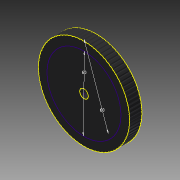
# Autodesk Inventor part: wheel 1
Saved by Autodesk Inventor 2014 (Build 180170000, 170)
## iProperties
Created: 2014-11-30
Part Number: wheel 1
Material: Generic
Document SubType Name: Modeling
Designer: ph1140784
Density: 1 g/cm^3
Appearance: Rubber - Black
Mass: 42.4685 g
Surface Area: 111.398 cm^2
Volume: 42.4685 cm^3
d0: 74.000 mm
d1: 10.000 mm
d2: 0.00 deg
d3: 7.000 mm
d4: 10.000 mm
d5: 0.00 deg
d7: 10.000 mm
d8: 0.00 deg
d9: 80.000 ul
d10: 360.00 deg
Author: ph1140784
Autodesk Inventor part; units mm, degrees
ref_plane "YZ Plane" through (0, 0, 0) normal (1, 0, 0) x (0, 1, 0)
ref_plane "XZ Plane" through (0, 0, 0) normal (0, 1, 0) x (-1, 0, 0)
ref_plane "XY Plane" through (0, 0, 0) normal (0, 0, 1) x (1, 0, 0)
sketch "Sketch1" plane through (0, 0, 0) normal (0, 1, 0) x (-1, 0, 0)
  circle A0 centre (0, 0) radius 37
  dimension "d0" = 74
  constraints: 1 centre point, 1 coincident
  measures "d0" diameter of A0
extrude "Extrusion1" add sketch "Sketch1" along normal blind 10
sketch "Sketch2" plane through (0, 10, 0) normal (0, 1, 0) x (1, 0, 0)
  circle A0 centre (0, 0) radius 37 projected
  circle A1 centre (0, 0) radius 3.5
  dimension "d3" = 7
  constraints: 1 centre point, 1 coincident
  measures "d3" diameter of A1
extrude "Extrusion2" cut sketch "Sketch2" against normal blind 10 contours A1
sketch "Sketch3" plane through (0, 10, 0) normal (0, 1, 0) x (1, 0, 0)
  circle A0 centre (0, 0) radius 37 projected
  line L0 (-16.7028, 33.0154) -> (-16.0314, 33.0154)
  line L1 (-16.0314, 33.0154) -> (-15.5404, 33.5782)
  constraints: 4 end point, 2 point on circle, 1 horizontal
extrude "Extrusion3" cut sketch "Sketch3" against normal blind 10 contours L1 L0 A0 picked at (-15.8339, 33.3296)
pattern_circular "Circular Pattern1" count 80 over 360 about axis through (0, -10, 0) along (0, 1, 0) of "Extrusion3"
sketch "Sketch4" plane through (0, 0, 0) normal (0, -1, 0) x (1, 0, 0)
  line L0 (-13.3916, -34.1714) -> (-12.858, -34.694) projected
  arc A0 (-12.858, -34.694) -> (-11.3324, -35.2218) centre (0, 0) ccw projected
  line L1 (-11.3324, -35.2218) -> (-10.6693, -35.1168) projected
  line L2 (-10.6693, -35.1168) -> (-10.0963, -35.5958) projected
  arc A1 (-10.0963, -35.5958) -> (-8.534, -36.0024) centre (0, 0) ccw projected
  line L3 (-8.534, -36.0024) -> (-7.8812, -35.8456) projected
  line L4 (-7.8812, -35.8456) -> (-7.2724, -36.2783) projected
  arc A2 (-7.2724, -36.2783) -> (-5.683, -36.561) centre (0, 0) ccw projected
  line L5 (-5.683, -36.561) -> (-5.0445, -36.3535) projected
  line L6 (-5.0445, -36.3535) -> (-4.4036, -36.737) projected
  arc A3 (-4.4036, -36.737) -> (-2.797, -36.8941) centre (0, 0) ccw projected
  line L7 (-2.797, -36.8941) -> (-2.1767, -36.6372) projected
  line L8 (-2.1767, -36.6372) -> (-1.5077, -36.9693) projected
  arc A4 (-1.5077, -36.9693) -> (0.1063, -36.9998) centre (0, 0) ccw projected
  line L9 (0.1063, -36.9998) -> (0.7046, -36.695) projected
  line L10 (0.7046, -36.695) -> (1.3976, -36.9736) projected
  arc A5 (1.3976, -36.9736) -> (3.009, -36.8774) centre (0, 0) ccw projected
  line L11 (3.009, -36.8774) -> (3.5815, -36.5266) projected
  line L12 (3.5815, -36.5266) -> (4.2942, -36.75) projected
  arc A6 (4.2942, -36.75) -> (5.8931, -36.5277) centre (0, 0) ccw projected
  line L13 (5.8931, -36.5277) -> (6.4363, -36.133) projected
  line L14 (6.4363, -36.133) -> (7.1643, -36.2998) projected
  arc A7 (7.1643, -36.2998) -> (8.7408, -35.9527) centre (0, 0) ccw projected
  line L15 (8.7408, -35.9527) -> (9.2514, -35.5167) projected
  line L16 (9.2514, -35.5167) -> (9.9903, -35.6258) projected
  arc A8 (9.9903, -35.6258) -> (11.5347, -35.1561) centre (0, 0) ccw projected
  line L17 (11.5347, -35.1561) -> (12.0095, -34.6813) projected
  line L18 (12.0095, -34.6813) -> (12.7546, -34.7321) projected
  arc A9 (12.7546, -34.7321) -> (14.2575, -34.1427) centre (0, 0) ccw projected
  line L19 (14.2575, -34.1427) -> (14.6935, -33.6322) projected
  line L20 (14.6935, -33.6322) -> (15.4404, -33.6243) projected
  arc A10 (15.4404, -33.6243) -> (16.8923, -32.9188) centre (0, 0) ccw projected
  line L21 (16.8923, -32.9188) -> (17.287, -32.3757) projected
  line L22 (17.287, -32.3757) -> (18.0309, -32.3092) projected
  arc A11 (18.0309, -32.3092) -> (19.423, -31.492) centre (0, 0) ccw projected
  line L23 (19.423, -31.492) -> (19.7738, -30.9195) projected
  line L24 (19.7738, -30.9195) -> (20.5103, -30.795) projected
  arc A12 (20.5103, -30.795) -> (21.834, -29.871) centre (0, 0) ccw projected
  line L25 (21.834, -29.871) -> (22.1388, -29.2728) projected
  line L26 (22.1388, -29.2728) -> (22.8632, -29.0908) projected
  arc A13 (22.8632, -29.0908) -> (24.1103, -28.0658) centre (0, 0) ccw projected
  line L27 (24.1103, -28.0658) -> (24.3673, -27.4455) projected
  line L28 (24.3673, -27.4455) -> (25.0751, -27.2073) projected
  arc A14 (25.0751, -27.2073) -> (26.238, -26.0876) centre (0, 0) ccw projected
  line L29 (26.238, -26.0876) -> (26.4455, -25.4491) projected
  line L30 (26.4455, -25.4491) -> (27.1325, -25.1561) projected
  arc A15 (27.1325, -25.1561) -> (28.204, -23.9486) centre (0, 0) ccw projected
  line L31 (28.204, -23.9486) -> (28.3607, -23.2958) projected
  line L32 (28.3607, -23.2958) -> (29.0226, -22.9497) projected
  arc A16 (29.0226, -22.9497) -> (29.996, -21.6619) centre (0, 0) ccw projected
  line L33 (29.996, -21.6619) -> (30.101, -20.9988) projected
  line L34 (30.101, -20.9988) -> (30.7337, -20.6019) projected
  arc A17 (30.7337, -20.6019) -> (31.6031, -19.2417) centre (0, 0) ccw projected
  line L35 (31.6031, -19.2417) -> (31.6558, -18.5724) projected
  line L36 (31.6558, -18.5724) -> (32.2554, -18.127) projected
  arc A18 (32.2554, -18.127) -> (33.0154, -16.7028) centre (0, 0) ccw projected
  line L37 (33.0154, -16.7028) -> (33.0154, -16.0314) projected
  line L38 (33.0154, -16.0314) -> (33.5782, -15.5404) projected
  arc A19 (33.5782, -15.5404) -> (34.2241, -14.061) centre (0, 0) ccw projected
  line L39 (34.2241, -14.061) -> (34.1714, -13.3916) projected
  line L40 (34.1714, -13.3916) -> (34.694, -12.858) projected
  arc A20 (34.694, -12.858) -> (35.2218, -11.3324) centre (0, 0) ccw projected
  line L41 (35.2218, -11.3324) -> (35.1168, -10.6693) projected
  line L42 (35.1168, -10.6693) -> (35.5958, -10.0963) projected
  arc A21 (35.5958, -10.0963) -> (36.0024, -8.534) centre (0, 0) ccw projected
  line L43 (36.0024, -8.534) -> (35.8456, -7.8812) projected
  line L44 (35.8456, -7.8812) -> (36.2783, -7.2724) projected
  arc A22 (36.2783, -7.2724) -> (36.561, -5.683) centre (0, 0) ccw projected
  line L45 (36.561, -5.683) -> (36.3535, -5.0445) projected
  line L46 (36.3535, -5.0445) -> (36.737, -4.4036) projected
  arc A23 (36.737, -4.4036) -> (36.8941, -2.797) centre (0, 0) ccw projected
  line L47 (36.8941, -2.797) -> (36.6372, -2.1767) projected
  line L48 (36.6372, -2.1767) -> (36.9693, -1.5077) projected
  arc A24 (36.9693, -1.5077) -> (36.9998, 0.1063) centre (0, 0) ccw projected
  line L49 (36.9998, 0.1063) -> (36.695, 0.7046) projected
  line L50 (36.695, 0.7046) -> (36.9736, 1.3976) projected
  arc A25 (36.9736, 1.3976) -> (36.8774, 3.009) centre (0, 0) ccw projected
  line L51 (36.8774, 3.009) -> (36.5266, 3.5815) projected
  line L52 (36.5266, 3.5815) -> (36.75, 4.2942) projected
  arc A26 (36.75, 4.2942) -> (36.5277, 5.8931) centre (0, 0) ccw projected
  line L53 (36.5277, 5.8931) -> (36.133, 6.4363) projected
  line L54 (36.133, 6.4363) -> (36.2998, 7.1643) projected
  arc A27 (36.2998, 7.1643) -> (35.9527, 8.7408) centre (0, 0) ccw projected
  line L55 (35.9527, 8.7408) -> (35.5167, 9.2514) projected
  line L56 (35.5167, 9.2514) -> (35.6258, 9.9903) projected
  arc A28 (35.6258, 9.9903) -> (35.1561, 11.5347) centre (0, 0) ccw projected
  line L57 (35.1561, 11.5347) -> (34.6813, 12.0095) projected
  line L58 (34.6813, 12.0095) -> (34.7321, 12.7546) projected
  arc A29 (34.7321, 12.7546) -> (34.1427, 14.2575) centre (0, 0) ccw projected
  line L59 (34.1427, 14.2575) -> (33.6322, 14.6935) projected
  line L60 (33.6322, 14.6935) -> (33.6243, 15.4404) projected
  arc A30 (33.6243, 15.4404) -> (32.9188, 16.8923) centre (0, 0) ccw projected
  line L61 (32.9188, 16.8923) -> (32.3757, 17.287) projected
  line L62 (32.3757, 17.287) -> (32.3092, 18.0309) projected
  arc A31 (32.3092, 18.0309) -> (31.492, 19.423) centre (0, 0) ccw projected
  line L63 (31.492, 19.423) -> (30.9195, 19.7738) projected
  line L64 (30.9195, 19.7738) -> (30.795, 20.5103) projected
  arc A32 (30.795, 20.5103) -> (29.871, 21.834) centre (0, 0) ccw projected
  line L65 (29.871, 21.834) -> (29.2728, 22.1388) projected
  line L66 (29.2728, 22.1388) -> (29.0908, 22.8632) projected
  arc A33 (29.0908, 22.8632) -> (28.0658, 24.1103) centre (0, 0) ccw projected
  line L67 (28.0658, 24.1103) -> (27.4455, 24.3673) projected
  line L68 (27.4455, 24.3673) -> (27.2073, 25.0751) projected
  arc A34 (27.2073, 25.0751) -> (26.0876, 26.238) centre (0, 0) ccw projected
  line L69 (26.0876, 26.238) -> (25.4491, 26.4455) projected
  line L70 (25.4491, 26.4455) -> (25.1561, 27.1325) projected
  arc A35 (25.1561, 27.1325) -> (23.9486, 28.204) centre (0, 0) ccw projected
  line L71 (23.9486, 28.204) -> (23.2958, 28.3607) projected
  line L72 (23.2958, 28.3607) -> (22.9497, 29.0226) projected
  arc A36 (22.9497, 29.0226) -> (21.6619, 29.996) centre (0, 0) ccw projected
  line L73 (21.6619, 29.996) -> (20.9988, 30.101) projected
  line L74 (20.9988, 30.101) -> (20.6019, 30.7337) projected
  arc A37 (20.6019, 30.7337) -> (19.2417, 31.6031) centre (0, 0) ccw projected
  line L75 (19.2417, 31.6031) -> (18.5724, 31.6558) projected
  line L76 (18.5724, 31.6558) -> (18.127, 32.2554) projected
  arc A38 (18.127, 32.2554) -> (16.7028, 33.0154) centre (0, 0) ccw projected
  line L77 (16.7028, 33.0154) -> (16.0314, 33.0154) projected
  line L78 (16.0314, 33.0154) -> (15.5404, 33.5782) projected
  arc A39 (15.5404, 33.5782) -> (14.061, 34.2241) centre (0, 0) ccw projected
  line L79 (14.061, 34.2241) -> (13.3916, 34.1714) projected
  line L80 (13.3916, 34.1714) -> (12.858, 34.694) projected
  arc A40 (12.858, 34.694) -> (11.3324, 35.2218) centre (0, 0) ccw projected
  line L81 (11.3324, 35.2218) -> (10.6693, 35.1168) projected
  line L82 (10.6693, 35.1168) -> (10.0963, 35.5958) projected
  arc A41 (10.0963, 35.5958) -> (8.534, 36.0024) centre (0, 0) ccw projected
  line L83 (8.534, 36.0024) -> (7.8812, 35.8456) projected
  line L84 (7.8812, 35.8456) -> (7.2724, 36.2783) projected
  arc A42 (7.2724, 36.2783) -> (5.683, 36.561) centre (0, 0) ccw projected
  line L85 (5.683, 36.561) -> (5.0445, 36.3535) projected
  line L86 (5.0445, 36.3535) -> (4.4036, 36.737) projected
  arc A43 (4.4036, 36.737) -> (2.797, 36.8941) centre (0, 0) ccw projected
  line L87 (2.797, 36.8941) -> (2.1767, 36.6372) projected
  line L88 (2.1767, 36.6372) -> (1.5077, 36.9693) projected
  arc A44 (1.5077, 36.9693) -> (-0.1063, 36.9998) centre (0, 0) ccw projected
  line L89 (-0.1063, 36.9998) -> (-0.7046, 36.695) projected
  line L90 (-0.7046, 36.695) -> (-1.3976, 36.9736) projected
  arc A45 (-1.3976, 36.9736) -> (-3.009, 36.8774) centre (0, 0) ccw projected
  line L91 (-3.009, 36.8774) -> (-3.5815, 36.5266) projected
  line L92 (-3.5815, 36.5266) -> (-4.2942, 36.75) projected
  arc A46 (-4.2942, 36.75) -> (-5.8931, 36.5277) centre (0, 0) ccw projected
  line L93 (-5.8931, 36.5277) -> (-6.4363, 36.133) projected
  line L94 (-6.4363, 36.133) -> (-7.1643, 36.2998) projected
  arc A47 (-7.1643, 36.2998) -> (-8.7408, 35.9527) centre (0, 0) ccw projected
  line L95 (-8.7408, 35.9527) -> (-9.2514, 35.5167) projected
  line L96 (-9.2514, 35.5167) -> (-9.9903, 35.6258) projected
  arc A48 (-9.9903, 35.6258) -> (-11.5347, 35.1561) centre (0, 0) ccw projected
  line L97 (-11.5347, 35.1561) -> (-12.0095, 34.6813) projected
  line L98 (-12.0095, 34.6813) -> (-12.7546, 34.7321) projected
  arc A49 (-12.7546, 34.7321) -> (-14.2575, 34.1427) centre (0, 0) ccw projected
  line L99 (-14.2575, 34.1427) -> (-14.6935, 33.6322) projected
  line L100 (-14.6935, 33.6322) -> (-15.4404, 33.6243) projected
  arc A50 (-15.4404, 33.6243) -> (-16.8923, 32.9188) centre (0, 0) ccw projected
  line L101 (-16.8923, 32.9188) -> (-17.287, 32.3757) projected
  line L102 (-17.287, 32.3757) -> (-18.0309, 32.3092) projected
  arc A51 (-18.0309, 32.3092) -> (-19.423, 31.492) centre (0, 0) ccw projected
  line L103 (-19.423, 31.492) -> (-19.7738, 30.9195) projected
  line L104 (-19.7738, 30.9195) -> (-20.5103, 30.795) projected
  arc A52 (-20.5103, 30.795) -> (-21.834, 29.871) centre (0, 0) ccw projected
  line L105 (-21.834, 29.871) -> (-22.1388, 29.2728) projected
  line L106 (-22.1388, 29.2728) -> (-22.8632, 29.0908) projected
  arc A53 (-22.8632, 29.0908) -> (-24.1103, 28.0658) centre (0, 0) ccw projected
  line L107 (-24.1103, 28.0658) -> (-24.3673, 27.4455) projected
  line L108 (-24.3673, 27.4455) -> (-25.0751, 27.2073) projected
  arc A54 (-25.0751, 27.2073) -> (-26.238, 26.0876) centre (0, 0) ccw projected
  line L109 (-26.238, 26.0876) -> (-26.4455, 25.4491) projected
  line L110 (-26.4455, 25.4491) -> (-27.1325, 25.1561) projected
  arc A55 (-27.1325, 25.1561) -> (-28.204, 23.9486) centre (0, 0) ccw projected
  line L111 (-28.204, 23.9486) -> (-28.3607, 23.2958) projected
  line L112 (-28.3607, 23.2958) -> (-29.0226, 22.9497) projected
  arc A56 (-29.0226, 22.9497) -> (-29.996, 21.6619) centre (0, 0) ccw projected
  line L113 (-29.996, 21.6619) -> (-30.101, 20.9988) projected
  line L114 (-30.101, 20.9988) -> (-30.7337, 20.6019) projected
  arc A57 (-30.7337, 20.6019) -> (-31.6031, 19.2417) centre (0, 0) ccw projected
  line L115 (-31.6031, 19.2417) -> (-31.6558, 18.5724) projected
  line L116 (-31.6558, 18.5724) -> (-32.2554, 18.127) projected
  arc A58 (-32.2554, 18.127) -> (-33.0154, 16.7028) centre (0, 0) ccw projected
  line L117 (-33.0154, 16.7028) -> (-33.0154, 16.0314) projected
  line L118 (-33.0154, 16.0314) -> (-33.5782, 15.5404) projected
  arc A59 (-33.5782, 15.5404) -> (-34.2241, 14.061) centre (0, 0) ccw projected
  line L119 (-34.2241, 14.061) -> (-34.1714, 13.3916) projected
  line L120 (-34.1714, 13.3916) -> (-34.694, 12.858) projected
  arc A60 (-34.694, 12.858) -> (-35.2218, 11.3324) centre (0, 0) ccw projected
  line L121 (-35.2218, 11.3324) -> (-35.1168, 10.6693) projected
  line L122 (-35.1168, 10.6693) -> (-35.5958, 10.0963) projected
  arc A61 (-35.5958, 10.0963) -> (-36.0024, 8.534) centre (0, 0) ccw projected
  line L123 (-36.0024, 8.534) -> (-35.8456, 7.8812) projected
  line L124 (-35.8456, 7.8812) -> (-36.2783, 7.2724) projected
  arc A62 (-36.2783, 7.2724) -> (-36.561, 5.683) centre (0, 0) ccw projected
  line L125 (-36.561, 5.683) -> (-36.3535, 5.0445) projected
  line L126 (-36.3535, 5.0445) -> (-36.737, 4.4036) projected
  arc A63 (-36.737, 4.4036) -> (-36.8941, 2.797) centre (0, 0) ccw projected
  line L127 (-36.8941, 2.797) -> (-36.6372, 2.1767) projected
  line L128 (-36.6372, 2.1767) -> (-36.9693, 1.5077) projected
  arc A64 (-36.9693, 1.5077) -> (-36.9998, -0.1063) centre (0, 0) ccw projected
  line L129 (-36.9998, -0.1063) -> (-36.695, -0.7046) projected
  line L130 (-36.695, -0.7046) -> (-36.9736, -1.3976) projected
  arc A65 (-36.9736, -1.3976) -> (-36.8774, -3.009) centre (0, 0) ccw projected
  line L131 (-36.8774, -3.009) -> (-36.5266, -3.5815) projected
  line L132 (-36.5266, -3.5815) -> (-36.75, -4.2942) projected
  arc A66 (-36.75, -4.2942) -> (-36.5277, -5.8931) centre (0, 0) ccw projected
  line L133 (-36.5277, -5.8931) -> (-36.133, -6.4363) projected
  line L134 (-36.133, -6.4363) -> (-36.2998, -7.1643) projected
  arc A67 (-36.2998, -7.1643) -> (-35.9527, -8.7408) centre (0, 0) ccw projected
  line L135 (-35.9527, -8.7408) -> (-35.5167, -9.2514) projected
  line L136 (-35.5167, -9.2514) -> (-35.6258, -9.9903) projected
  arc A68 (-35.6258, -9.9903) -> (-35.1561, -11.5347) centre (0, 0) ccw projected
  line L137 (-35.1561, -11.5347) -> (-34.6813, -12.0095) projected
  line L138 (-34.6813, -12.0095) -> (-34.7321, -12.7546) projected
  arc A69 (-34.7321, -12.7546) -> (-34.1427, -14.2575) centre (0, 0) ccw projected
  line L139 (-34.1427, -14.2575) -> (-33.6322, -14.6935) projected
  line L140 (-33.6322, -14.6935) -> (-33.6243, -15.4404) projected
  arc A70 (-33.6243, -15.4404) -> (-32.9188, -16.8923) centre (0, 0) ccw projected
  line L141 (-32.9188, -16.8923) -> (-32.3757, -17.287) projected
  line L142 (-32.3757, -17.287) -> (-32.3092, -18.0309) projected
  arc A71 (-32.3092, -18.0309) -> (-31.492, -19.423) centre (0, 0) ccw projected
  line L143 (-31.492, -19.423) -> (-30.9195, -19.7738) projected
  line L144 (-30.9195, -19.7738) -> (-30.795, -20.5103) projected
  arc A72 (-30.795, -20.5103) -> (-29.871, -21.834) centre (0, 0) ccw projected
  line L145 (-29.871, -21.834) -> (-29.2728, -22.1388) projected
  line L146 (-29.2728, -22.1388) -> (-29.0908, -22.8632) projected
  arc A73 (-29.0908, -22.8632) -> (-28.0658, -24.1103) centre (0, 0) ccw projected
  line L147 (-28.0658, -24.1103) -> (-27.4455, -24.3673) projected
  line L148 (-27.4455, -24.3673) -> (-27.2073, -25.0751) projected
  arc A74 (-27.2073, -25.0751) -> (-26.0876, -26.238) centre (0, 0) ccw projected
  line L149 (-26.0876, -26.238) -> (-25.4491, -26.4455) projected
  line L150 (-25.4491, -26.4455) -> (-25.1561, -27.1325) projected
  arc A75 (-25.1561, -27.1325) -> (-23.9486, -28.204) centre (0, 0) ccw projected
  line L151 (-23.9486, -28.204) -> (-23.2958, -28.3607) projected
  line L152 (-23.2958, -28.3607) -> (-22.9497, -29.0226) projected
  arc A76 (-22.9497, -29.0226) -> (-21.6619, -29.996) centre (0, 0) ccw projected
  line L153 (-21.6619, -29.996) -> (-20.9988, -30.101) projected
  line L154 (-20.9988, -30.101) -> (-20.6019, -30.7337) projected
  arc A77 (-20.6019, -30.7337) -> (-19.2417, -31.6031) centre (0, 0) ccw projected
  line L155 (-19.2417, -31.6031) -> (-18.5724, -31.6558) projected
  line L156 (-18.5724, -31.6558) -> (-18.127, -32.2554) projected
  arc A78 (-18.127, -32.2554) -> (-16.7028, -33.0154) centre (0, 0) ccw projected
  line L157 (-16.7028, -33.0154) -> (-16.0314, -33.0154) projected
  line L158 (-16.0314, -33.0154) -> (-15.5404, -33.5782) projected
  arc A79 (-15.5404, -33.5782) -> (-14.061, -34.2241) centre (0, 0) ccw projected
  line L159 (-14.061, -34.2241) -> (-13.3916, -34.1714) projected
  circle A80 centre (0, 0) radius 3.5 projected
  circle A81 centre (0, 0) radius 30
  dimension "d12" = 60
  constraints: 1 centre point, 1 coincident
  measures "d12" diameter of A81
sketch "Sketch5" plane through (0, 10, 0) normal (0, 1, 0) x (1, 0, 0)
  circle A0 centre (0, 0) radius 3.5 projected
  line L0 (-12.858, 34.694) -> (-13.3916, 34.1714) projected
  line L1 (-13.3916, 34.1714) -> (-14.061, 34.2241) projected
  arc A1 (-14.061, 34.2241) -> (-15.5404, 33.5782) centre (0, 0) ccw projected
  line L2 (-15.5404, 33.5782) -> (-16.0314, 33.0154) projected
  line L3 (-16.0314, 33.0154) -> (-16.7028, 33.0154) projected
  arc A2 (-16.7028, 33.0154) -> (-18.127, 32.2554) centre (0, 0) ccw projected
  line L4 (-18.127, 32.2554) -> (-18.5724, 31.6558) projected
  line L5 (-18.5724, 31.6558) -> (-19.2417, 31.6031) projected
  arc A3 (-19.2417, 31.6031) -> (-20.6019, 30.7337) centre (0, 0) ccw projected
  line L6 (-20.6019, 30.7337) -> (-20.9988, 30.101) projected
  line L7 (-20.9988, 30.101) -> (-21.6619, 29.996) projected
  arc A4 (-21.6619, 29.996) -> (-22.9497, 29.0226) centre (0, 0) ccw projected
  line L8 (-22.9497, 29.0226) -> (-23.2958, 28.3607) projected
  line L9 (-23.2958, 28.3607) -> (-23.9486, 28.204) projected
  arc A5 (-23.9486, 28.204) -> (-25.1561, 27.1325) centre (0, 0) ccw projected
  line L10 (-25.1561, 27.1325) -> (-25.4491, 26.4455) projected
  line L11 (-25.4491, 26.4455) -> (-26.0876, 26.238) projected
  arc A6 (-26.0876, 26.238) -> (-27.2073, 25.0751) centre (0, 0) ccw projected
  line L12 (-27.2073, 25.0751) -> (-27.4455, 24.3673) projected
  line L13 (-27.4455, 24.3673) -> (-28.0658, 24.1103) projected
  arc A7 (-28.0658, 24.1103) -> (-29.0908, 22.8632) centre (0, 0) ccw projected
  line L14 (-29.0908, 22.8632) -> (-29.2728, 22.1388) projected
  line L15 (-29.2728, 22.1388) -> (-29.871, 21.834) projected
  arc A8 (-29.871, 21.834) -> (-30.795, 20.5103) centre (0, 0) ccw projected
  line L16 (-30.795, 20.5103) -> (-30.9195, 19.7738) projected
  line L17 (-30.9195, 19.7738) -> (-31.492, 19.423) projected
  arc A9 (-31.492, 19.423) -> (-32.3092, 18.0309) centre (0, 0) ccw projected
  line L18 (-32.3092, 18.0309) -> (-32.3757, 17.287) projected
  line L19 (-32.3757, 17.287) -> (-32.9188, 16.8923) projected
  arc A10 (-32.9188, 16.8923) -> (-33.6243, 15.4404) centre (0, 0) ccw projected
  line L20 (-33.6243, 15.4404) -> (-33.6322, 14.6935) projected
  line L21 (-33.6322, 14.6935) -> (-34.1427, 14.2575) projected
  arc A11 (-34.1427, 14.2575) -> (-34.7321, 12.7546) centre (0, 0) ccw projected
  line L22 (-34.7321, 12.7546) -> (-34.6813, 12.0095) projected
  line L23 (-34.6813, 12.0095) -> (-35.1561, 11.5347) projected
  arc A12 (-35.1561, 11.5347) -> (-35.6258, 9.9903) centre (0, 0) ccw projected
  line L24 (-35.6258, 9.9903) -> (-35.5167, 9.2514) projected
  line L25 (-35.5167, 9.2514) -> (-35.9527, 8.7408) projected
  arc A13 (-35.9527, 8.7408) -> (-36.2998, 7.1643) centre (0, 0) ccw projected
  line L26 (-36.2998, 7.1643) -> (-36.133, 6.4363) projected
  line L27 (-36.133, 6.4363) -> (-36.5277, 5.8931) projected
  arc A14 (-36.5277, 5.8931) -> (-36.75, 4.2942) centre (0, 0) ccw projected
  line L28 (-36.75, 4.2942) -> (-36.5266, 3.5815) projected
  line L29 (-36.5266, 3.5815) -> (-36.8774, 3.009) projected
  arc A15 (-36.8774, 3.009) -> (-36.9736, 1.3976) centre (0, 0) ccw projected
  line L30 (-36.9736, 1.3976) -> (-36.695, 0.7046) projected
  line L31 (-36.695, 0.7046) -> (-36.9998, 0.1063) projected
  arc A16 (-36.9998, 0.1063) -> (-36.9693, -1.5077) centre (0, 0) ccw projected
  line L32 (-36.9693, -1.5077) -> (-36.6372, -2.1767) projected
  line L33 (-36.6372, -2.1767) -> (-36.8941, -2.797) projected
  arc A17 (-36.8941, -2.797) -> (-36.737, -4.4036) centre (0, 0) ccw projected
  line L34 (-36.737, -4.4036) -> (-36.3535, -5.0445) projected
  line L35 (-36.3535, -5.0445) -> (-36.561, -5.683) projected
  arc A18 (-36.561, -5.683) -> (-36.2783, -7.2724) centre (0, 0) ccw projected
  line L36 (-36.2783, -7.2724) -> (-35.8456, -7.8812) projected
  line L37 (-35.8456, -7.8812) -> (-36.0024, -8.534) projected
  arc A19 (-36.0024, -8.534) -> (-35.5958, -10.0963) centre (0, 0) ccw projected
  line L38 (-35.5958, -10.0963) -> (-35.1168, -10.6693) projected
  line L39 (-35.1168, -10.6693) -> (-35.2218, -11.3324) projected
  arc A20 (-35.2218, -11.3324) -> (-34.694, -12.858) centre (0, 0) ccw projected
  line L40 (-34.694, -12.858) -> (-34.1714, -13.3916) projected
  line L41 (-34.1714, -13.3916) -> (-34.2241, -14.061) projected
  arc A21 (-34.2241, -14.061) -> (-33.5782, -15.5404) centre (0, 0) ccw projected
  line L42 (-33.5782, -15.5404) -> (-33.0154, -16.0314) projected
  line L43 (-33.0154, -16.0314) -> (-33.0154, -16.7028) projected
  arc A22 (-33.0154, -16.7028) -> (-32.2554, -18.127) centre (0, 0) ccw projected
  line L44 (-32.2554, -18.127) -> (-31.6558, -18.5724) projected
  line L45 (-31.6558, -18.5724) -> (-31.6031, -19.2417) projected
  arc A23 (-31.6031, -19.2417) -> (-30.7337, -20.6019) centre (0, 0) ccw projected
  line L46 (-30.7337, -20.6019) -> (-30.101, -20.9988) projected
  line L47 (-30.101, -20.9988) -> (-29.996, -21.6619) projected
  arc A24 (-29.996, -21.6619) -> (-29.0226, -22.9497) centre (0, 0) ccw projected
  line L48 (-29.0226, -22.9497) -> (-28.3607, -23.2958) projected
  line L49 (-28.3607, -23.2958) -> (-28.204, -23.9486) projected
  arc A25 (-28.204, -23.9486) -> (-27.1325, -25.1561) centre (0, 0) ccw projected
  line L50 (-27.1325, -25.1561) -> (-26.4455, -25.4491) projected
  line L51 (-26.4455, -25.4491) -> (-26.238, -26.0876) projected
  arc A26 (-26.238, -26.0876) -> (-25.0751, -27.2073) centre (0, 0) ccw projected
  line L52 (-25.0751, -27.2073) -> (-24.3673, -27.4455) projected
  line L53 (-24.3673, -27.4455) -> (-24.1103, -28.0658) projected
  arc A27 (-24.1103, -28.0658) -> (-22.8632, -29.0908) centre (0, 0) ccw projected
  line L54 (-22.8632, -29.0908) -> (-22.1388, -29.2728) projected
  line L55 (-22.1388, -29.2728) -> (-21.834, -29.871) projected
  arc A28 (-21.834, -29.871) -> (-20.5103, -30.795) centre (0, 0) ccw projected
  line L56 (-20.5103, -30.795) -> (-19.7738, -30.9195) projected
  line L57 (-19.7738, -30.9195) -> (-19.423, -31.492) projected
  arc A29 (-19.423, -31.492) -> (-18.0309, -32.3092) centre (0, 0) ccw projected
  line L58 (-18.0309, -32.3092) -> (-17.287, -32.3757) projected
  line L59 (-17.287, -32.3757) -> (-16.8923, -32.9188) projected
  arc A30 (-16.8923, -32.9188) -> (-15.4404, -33.6243) centre (0, 0) ccw projected
  line L60 (-15.4404, -33.6243) -> (-14.6935, -33.6322) projected
  line L61 (-14.6935, -33.6322) -> (-14.2575, -34.1427) projected
  arc A31 (-14.2575, -34.1427) -> (-12.7546, -34.7321) centre (0, 0) ccw projected
  line L62 (-12.7546, -34.7321) -> (-12.0095, -34.6813) projected
  line L63 (-12.0095, -34.6813) -> (-11.5347, -35.1561) projected
  arc A32 (-11.5347, -35.1561) -> (-9.9903, -35.6258) centre (0, 0) ccw projected
  line L64 (-9.9903, -35.6258) -> (-9.2514, -35.5167) projected
  line L65 (-9.2514, -35.5167) -> (-8.7408, -35.9527) projected
  arc A33 (-8.7408, -35.9527) -> (-7.1643, -36.2998) centre (0, 0) ccw projected
  line L66 (-7.1643, -36.2998) -> (-6.4363, -36.133) projected
  line L67 (-6.4363, -36.133) -> (-5.8931, -36.5277) projected
  arc A34 (-5.8931, -36.5277) -> (-4.2942, -36.75) centre (0, 0) ccw projected
  line L68 (-4.2942, -36.75) -> (-3.5815, -36.5266) projected
  line L69 (-3.5815, -36.5266) -> (-3.009, -36.8774) projected
  arc A35 (-3.009, -36.8774) -> (-1.3976, -36.9736) centre (0, 0) ccw projected
  line L70 (-1.3976, -36.9736) -> (-0.7046, -36.695) projected
  line L71 (-0.7046, -36.695) -> (-0.1063, -36.9998) projected
  arc A36 (-0.1063, -36.9998) -> (1.5077, -36.9693) centre (0, 0) ccw projected
  line L72 (1.5077, -36.9693) -> (2.1767, -36.6372) projected
  line L73 (2.1767, -36.6372) -> (2.797, -36.8941) projected
  arc A37 (2.797, -36.8941) -> (4.4036, -36.737) centre (0, 0) ccw projected
  line L74 (4.4036, -36.737) -> (5.0445, -36.3535) projected
  line L75 (5.0445, -36.3535) -> (5.683, -36.561) projected
  arc A38 (5.683, -36.561) -> (7.2724, -36.2783) centre (0, 0) ccw projected
  line L76 (7.2724, -36.2783) -> (7.8812, -35.8456) projected
  line L77 (7.8812, -35.8456) -> (8.534, -36.0024) projected
  arc A39 (8.534, -36.0024) -> (10.0963, -35.5958) centre (0, 0) ccw projected
  line L78 (10.0963, -35.5958) -> (10.6693, -35.1168) projected
  line L79 (10.6693, -35.1168) -> (11.3324, -35.2218) projected
  arc A40 (11.3324, -35.2218) -> (12.858, -34.694) centre (0, 0) ccw projected
  line L80 (12.858, -34.694) -> (13.3916, -34.1714) projected
  line L81 (13.3916, -34.1714) -> (14.061, -34.2241) projected
  arc A41 (14.061, -34.2241) -> (15.5404, -33.5782) centre (0, 0) ccw projected
  line L82 (15.5404, -33.5782) -> (16.0314, -33.0154) projected
  line L83 (16.0314, -33.0154) -> (16.7028, -33.0154) projected
  arc A42 (16.7028, -33.0154) -> (18.127, -32.2554) centre (0, 0) ccw projected
  line L84 (18.127, -32.2554) -> (18.5724, -31.6558) projected
  line L85 (18.5724, -31.6558) -> (19.2417, -31.6031) projected
  arc A43 (19.2417, -31.6031) -> (20.6019, -30.7337) centre (0, 0) ccw projected
  line L86 (20.6019, -30.7337) -> (20.9988, -30.101) projected
  line L87 (20.9988, -30.101) -> (21.6619, -29.996) projected
  arc A44 (21.6619, -29.996) -> (22.9497, -29.0226) centre (0, 0) ccw projected
  line L88 (22.9497, -29.0226) -> (23.2958, -28.3607) projected
  line L89 (23.2958, -28.3607) -> (23.9486, -28.204) projected
  arc A45 (23.9486, -28.204) -> (25.1561, -27.1325) centre (0, 0) ccw projected
  line L90 (25.1561, -27.1325) -> (25.4491, -26.4455) projected
  line L91 (25.4491, -26.4455) -> (26.0876, -26.238) projected
  arc A46 (26.0876, -26.238) -> (27.2073, -25.0751) centre (0, 0) ccw projected
  line L92 (27.2073, -25.0751) -> (27.4455, -24.3673) projected
  line L93 (27.4455, -24.3673) -> (28.0658, -24.1103) projected
  arc A47 (28.0658, -24.1103) -> (29.0908, -22.8632) centre (0, 0) ccw projected
  line L94 (29.0908, -22.8632) -> (29.2728, -22.1388) projected
  line L95 (29.2728, -22.1388) -> (29.871, -21.834) projected
  arc A48 (29.871, -21.834) -> (30.795, -20.5103) centre (0, 0) ccw projected
  line L96 (30.795, -20.5103) -> (30.9195, -19.7738) projected
  line L97 (30.9195, -19.7738) -> (31.492, -19.423) projected
  arc A49 (31.492, -19.423) -> (32.3092, -18.0309) centre (0, 0) ccw projected
  line L98 (32.3092, -18.0309) -> (32.3757, -17.287) projected
  line L99 (32.3757, -17.287) -> (32.9188, -16.8923) projected
  arc A50 (32.9188, -16.8923) -> (33.6243, -15.4404) centre (0, 0) ccw projected
  line L100 (33.6243, -15.4404) -> (33.6322, -14.6935) projected
  line L101 (33.6322, -14.6935) -> (34.1427, -14.2575) projected
  arc A51 (34.1427, -14.2575) -> (34.7321, -12.7546) centre (0, 0) ccw projected
  line L102 (34.7321, -12.7546) -> (34.6813, -12.0095) projected
  line L103 (34.6813, -12.0095) -> (35.1561, -11.5347) projected
  arc A52 (35.1561, -11.5347) -> (35.6258, -9.9903) centre (0, 0) ccw projected
  line L104 (35.6258, -9.9903) -> (35.5167, -9.2514) projected
  line L105 (35.5167, -9.2514) -> (35.9527, -8.7408) projected
  arc A53 (35.9527, -8.7408) -> (36.2998, -7.1643) centre (0, 0) ccw projected
  line L106 (36.2998, -7.1643) -> (36.133, -6.4363) projected
  line L107 (36.133, -6.4363) -> (36.5277, -5.8931) projected
  arc A54 (36.5277, -5.8931) -> (36.75, -4.2942) centre (0, 0) ccw projected
  line L108 (36.75, -4.2942) -> (36.5266, -3.5815) projected
  line L109 (36.5266, -3.5815) -> (36.8774, -3.009) projected
  arc A55 (36.8774, -3.009) -> (36.9736, -1.3976) centre (0, 0) ccw projected
  line L110 (36.9736, -1.3976) -> (36.695, -0.7046) projected
  line L111 (36.695, -0.7046) -> (36.9998, -0.1063) projected
  arc A56 (36.9998, -0.1063) -> (36.9693, 1.5077) centre (0, 0) ccw projected
  line L112 (36.9693, 1.5077) -> (36.6372, 2.1767) projected
  line L113 (36.6372, 2.1767) -> (36.8941, 2.797) projected
  arc A57 (36.8941, 2.797) -> (36.737, 4.4036) centre (0, 0) ccw projected
  line L114 (36.737, 4.4036) -> (36.3535, 5.0445) projected
  line L115 (36.3535, 5.0445) -> (36.561, 5.683) projected
  arc A58 (36.561, 5.683) -> (36.2783, 7.2724) centre (0, 0) ccw projected
  line L116 (36.2783, 7.2724) -> (35.8456, 7.8812) projected
  line L117 (35.8456, 7.8812) -> (36.0024, 8.534) projected
  arc A59 (36.0024, 8.534) -> (35.5958, 10.0963) centre (0, 0) ccw projected
  line L118 (35.5958, 10.0963) -> (35.1168, 10.6693) projected
  line L119 (35.1168, 10.6693) -> (35.2218, 11.3324) projected
  arc A60 (35.2218, 11.3324) -> (34.694, 12.858) centre (0, 0) ccw projected
  line L120 (34.694, 12.858) -> (34.1714, 13.3916) projected
  line L121 (34.1714, 13.3916) -> (34.2241, 14.061) projected
  arc A61 (34.2241, 14.061) -> (33.5782, 15.5404) centre (0, 0) ccw projected
  line L122 (33.5782, 15.5404) -> (33.0154, 16.0314) projected
  line L123 (33.0154, 16.0314) -> (33.0154, 16.7028) projected
  arc A62 (33.0154, 16.7028) -> (32.2554, 18.127) centre (0, 0) ccw projected
  line L124 (32.2554, 18.127) -> (31.6558, 18.5724) projected
  line L125 (31.6558, 18.5724) -> (31.6031, 19.2417) projected
  arc A63 (31.6031, 19.2417) -> (30.7337, 20.6019) centre (0, 0) ccw projected
  line L126 (30.7337, 20.6019) -> (30.101, 20.9988) projected
  line L127 (30.101, 20.9988) -> (29.996, 21.6619) projected
  arc A64 (29.996, 21.6619) -> (29.0226, 22.9497) centre (0, 0) ccw projected
  line L128 (29.0226, 22.9497) -> (28.3607, 23.2958) projected
  line L129 (28.3607, 23.2958) -> (28.204, 23.9486) projected
  arc A65 (28.204, 23.9486) -> (27.1325, 25.1561) centre (0, 0) ccw projected
  line L130 (27.1325, 25.1561) -> (26.4455, 25.4491) projected
  line L131 (26.4455, 25.4491) -> (26.238, 26.0876) projected
  arc A66 (26.238, 26.0876) -> (25.0751, 27.2073) centre (0, 0) ccw projected
  line L132 (25.0751, 27.2073) -> (24.3673, 27.4455) projected
  line L133 (24.3673, 27.4455) -> (24.1103, 28.0658) projected
  arc A67 (24.1103, 28.0658) -> (22.8632, 29.0908) centre (0, 0) ccw projected
  line L134 (22.8632, 29.0908) -> (22.1388, 29.2728) projected
  line L135 (22.1388, 29.2728) -> (21.834, 29.871) projected
  arc A68 (21.834, 29.871) -> (20.5103, 30.795) centre (0, 0) ccw projected
  line L136 (20.5103, 30.795) -> (19.7738, 30.9195) projected
  line L137 (19.7738, 30.9195) -> (19.423, 31.492) projected
  arc A69 (19.423, 31.492) -> (18.0309, 32.3092) centre (0, 0) ccw projected
  line L138 (18.0309, 32.3092) -> (17.287, 32.3757) projected
  line L139 (17.287, 32.3757) -> (16.8923, 32.9188) projected
  arc A70 (16.8923, 32.9188) -> (15.4404, 33.6243) centre (0, 0) ccw projected
  line L140 (15.4404, 33.6243) -> (14.6935, 33.6322) projected
  line L141 (14.6935, 33.6322) -> (14.2575, 34.1427) projected
  arc A71 (14.2575, 34.1427) -> (12.7546, 34.7321) centre (0, 0) ccw projected
  line L142 (12.7546, 34.7321) -> (12.0095, 34.6813) projected
  line L143 (12.0095, 34.6813) -> (11.5347, 35.1561) projected
  arc A72 (11.5347, 35.1561) -> (9.9903, 35.6258) centre (0, 0) ccw projected
  line L144 (9.9903, 35.6258) -> (9.2514, 35.5167) projected
  line L145 (9.2514, 35.5167) -> (8.7408, 35.9527) projected
  arc A73 (8.7408, 35.9527) -> (7.1643, 36.2998) centre (0, 0) ccw projected
  line L146 (7.1643, 36.2998) -> (6.4363, 36.133) projected
  line L147 (6.4363, 36.133) -> (5.8931, 36.5277) projected
  arc A74 (5.8931, 36.5277) -> (4.2942, 36.75) centre (0, 0) ccw projected
  line L148 (4.2942, 36.75) -> (3.5815, 36.5266) projected
  line L149 (3.5815, 36.5266) -> (3.009, 36.8774) projected
  arc A75 (3.009, 36.8774) -> (1.3976, 36.9736) centre (0, 0) ccw projected
  line L150 (1.3976, 36.9736) -> (0.7046, 36.695) projected
  line L151 (0.7046, 36.695) -> (0.1063, 36.9998) projected
  arc A76 (0.1063, 36.9998) -> (-1.5077, 36.9693) centre (0, 0) ccw projected
  line L152 (-1.5077, 36.9693) -> (-2.1767, 36.6372) projected
  line L153 (-2.1767, 36.6372) -> (-2.797, 36.8941) projected
  arc A77 (-2.797, 36.8941) -> (-4.4036, 36.737) centre (0, 0) ccw projected
  line L154 (-4.4036, 36.737) -> (-5.0445, 36.3535) projected
  line L155 (-5.0445, 36.3535) -> (-5.683, 36.561) projected
  arc A78 (-5.683, 36.561) -> (-7.2724, 36.2783) centre (0, 0) ccw projected
  line L156 (-7.2724, 36.2783) -> (-7.8812, 35.8456) projected
  line L157 (-7.8812, 35.8456) -> (-8.534, 36.0024) projected
  arc A79 (-8.534, 36.0024) -> (-10.0963, 35.5958) centre (0, 0) ccw projected
  line L158 (-10.0963, 35.5958) -> (-10.6693, 35.1168) projected
  line L159 (-10.6693, 35.1168) -> (-11.3324, 35.2218) projected
  arc A80 (-11.3324, 35.2218) -> (-12.858, 34.694) centre (0, 0) ccw projected
  circle A81 centre (0, 0) radius 30
  dimension "d13" = 60
  constraints: 1 centre point, 1 coincident
  measures "d13" diameter of A81
body "Solid1"
